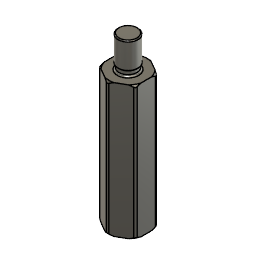
M3 Parametric M-F Standoff (Autodesk Fusion 360 design; units mm, degrees)
part number: 20-4 M-F Standoff
Autodesk Fusion 360 part; units mm, degrees
note: some values were not read from the file. Set by a fixed rule: which sketch regions a step uses.
sketch "M3 Standoff Profile" plane through (0, 0, 0) normal (0, 1, 0) x (1, 0, 0)
  arc A0 (-2.75, -1.3669) -> (-2.5588, -1.6981) centre (-2.3675, -1.3669) ccw
  arc A1 (0.1912, 3.065) -> (-0.1913, 3.065) centre (0, 2.7338) ccw
  arc A2 (-0.1912, -3.065) -> (0.1913, -3.065) centre (0, -2.7338) ccw
  arc A3 (2.5588, -1.6981) -> (2.75, -1.3669) centre (2.3675, -1.3669) ccw
  line L0 (2.75, -1.3669) -> (2.75, 1.3669)
  line L1 (-2.75, 1.3669) -> (-2.75, -1.3669)
  arc A4 (2.75, 1.3669) -> (2.5588, 1.6981) centre (2.3675, 1.3669) ccw
  line L2 (-0.1913, 3.065) -> (-2.5588, 1.6981)
  line L3 (2.5587, 1.6981) -> (0.1912, 3.065)
  line L4 (-2.5588, -1.6981) -> (-0.1912, -3.065)
  line L5 (0.1913, -3.065) -> (2.5588, -1.6981)
  arc A5 (-2.5588, 1.6981) -> (-2.75, 1.3669) centre (-2.3675, 1.3669) ccw
  line L6 (0, 2.7338) -> (0, -2.7338) construction
  dimension "d28" = 120
  dimension "d29" = 0.3825
  dimension "d30" = 2.75
  dimension "d31" = 5.5
  dimension "d32" = 120
  constraint equal A1 A4
  constraint equal A3 A4
  constraint equal A2 A3
  constraint equal A0 A2
  constraint equal A0 A5
  constraint tangent A1 L3
  constraint tangent A1 L2
  constraint tangent A4 L3
  constraint tangent L0 A4
  constraint tangent A3 L5
  constraint tangent A3 L0
  constraint tangent A2 L5
  constraint tangent A2 L4
  constraint tangent A0 L4
  constraint tangent A0 L1
  constraint tangent L1 A5
  constraint tangent L2 A5
  constraint equal L0 L5
  constraint equal L4 L5
  constraint equal L1 L5
  constraint equal L1 L2
  constraint equal L2 L3
  constraint vertical L0
  constraint coincident A1.centre L6.start
  constraint coincident A2.centre L6.end
  constraint midpoint origin L6
  measures "d28" angle of L0 L3
  measures "d29" radius of A5
  measures "d30" distance of origin L0
  measures "d31" distance of L0 L1
  measures "d32" angle of L2 L3
extrude "Extrude1" add sketch "M3 Standoff Profile" along normal blind 20
hole "Hole1" at (0, 0, 0) direction (0, 1, 0) diameter 2.529 depth 8 tip angle 118
thread "Thread1" "ISO Metric profile 3.0 M3x0.5 6H" thread offset 0 thread depth 7.4
ref_plane "WorkPlane1" through (0, 10, 0) normal (0.5, 0, 0.866025) x (0.866025, 0, -0.5)
sketch "Sketch2" plane through (0, 0, 0) normal (0.5, 0, 0.866025) x (0.866025, 0, -0.5)
  line L0 (-3.065, 0) -> (-1.6981, 0)
  line L1 (-1.6981, 0) -> (-1.6981, 20)
  line L2 (-1.6981, 20) -> (-3.065, 20)
  line L3 (-3.065, 20) -> (-3.065, 0)
  line L4 (1.6981, 0) -> (3.065, 0)
  line L5 (3.065, 20) -> (1.6981, 20)
  line L6 (1.6981, 20) -> (1.6981, 0)
  line L7 (-3.065, 0) -> (-3.1163, 0)
  line L8 (-3.065, 0) -> (-3.065, 20)
  line L9 (-3.065, 20) -> (-3.1163, 20)
  line L10 (-3.065, 20) -> (-3.065, 0)
  line L11 (3.1163, 0) -> (3.065, 0)
  line L12 (3.1163, 20) -> (3.065, 20)
  line L13 (3.065, 20) -> (3.065, 0) construction
  line L14 (1.6981, 0) -> (1.3669, 0)
  line L15 (1.6981, 0) -> (1.6981, 20)
  line L16 (1.6981, 20) -> (1.3669, 20)
  line L17 (1.3669, 20) -> (1.3669, 0)
  line L18 (3.1163, 0) -> (3.1163, 0.25)
  line L19 (3.1163, 0) -> (2.8663, 0)
  line L20 (2.8663, 0) -> (3.1163, 0.25)
  line L21 (3.1163, 20) -> (2.8663, 20)
  line L22 (3.1163, 20) -> (3.1163, 19.75)
  line L23 (2.8663, 20) -> (3.1163, 19.75)
  dimension "d12" = 0.25
  dimension "d13" = 0.25
  dimension "d14" = 0.25
  dimension "d15" = 0.25
  constraint coincident L11.start L18.start
  constraint perpendicular L11 L18
  constraint perpendicular L18 L19
  constraint coincident L12.start L21.start
  constraint perpendicular L12 L22
  constraint horizontal L21
  measures "d12" distance of L11.start L18.end
  measures "d13" distance of L11.start L19.end
  measures "d14" distance of L12.start L21.end
  measures "d15" distance of L12.start L22.end
revolve "Revolve1" cut sketch "Sketch2" angle 360 about axis through (0, 1.75, 0) along (0, 1, 0) contours L4 L11 L18 L19 L20 | L5 L12 L21 L22 L23
sketch "Sketch3" plane through (0, 20, 0) normal (0, 1, 0) x (-1, 0, 0)
  arc A0 (-0.6752, -2.7856) -> (0.6752, -2.7856) centre (0, 0) ccw
  line L0 (0.6752, -2.7856) -> (2.0748, -1.9776)
  arc A1 (2.0748, -1.9776) -> (2.75, -0.808) centre (0, 0) ccw
  line L1 (2.75, -0.808) -> (2.75, 0.808)
  arc A2 (2.75, 0.808) -> (2.0748, 1.9776) centre (0, 0) ccw
  line L2 (2.0748, 1.9776) -> (0.6752, 2.7856)
  arc A3 (0.6752, 2.7856) -> (-0.6752, 2.7856) centre (0, 0) ccw
  line L3 (-0.6752, 2.7856) -> (-2.0748, 1.9776)
  arc A4 (-2.0748, 1.9776) -> (-2.75, 0.808) centre (0, 0) ccw
  line L4 (-2.75, 0.808) -> (-2.75, -0.808)
  arc A5 (-2.75, -0.808) -> (-2.0748, -1.9776) centre (0, 0) ccw
  line L5 (-2.0748, -1.9776) -> (-0.6752, -2.7856)
  circle A6 centre (0, 0) radius 1.5
  circle A7 centre (0, 0) radius 1.35
  dimension "d17" = 3
  dimension "d18" = 2.7
  constraint concentric A0 A6
  constraint concentric A0 A7
  measures "d17" diameter of A6
  measures "d18" diameter of A7
extrude "Extrude2" add sketch "Sketch3" along normal blind 0.75 contours A7
extrude "Extrude3" add sketch "Sketch3" along normal blind 4 from surface at 0.75 contours A6 | A7
fillet "Fillet1" radius 0.25 1 edges at (1.2586, 20, 0.4882)
chamfer "Chamfer3" distance 0.15 angle 45 2 edges at (1.3985, 20.75, -0.5424) (1.3985, 24.75, -0.5424)
chamfer "Chamfer3" distance 0.3 angle 45 1 edges at (0.4573, 0, 1.1789)
equation "Thread_Length = 4 mm" comment "Thread Length"
equation "Spacing = 20 mm" comment "Standoff section"
equation "d3 = Spacing"
equation "d22 = Thread_Length"
equation "d30 = Hex_Width / 2"
equation "d31 = d30 * 2"
equation "d32 = d28"
equation "Hex_Width = 5.5 mm"
